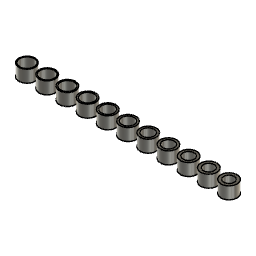
Smartphone inserts generator v4 (Autodesk Fusion 360 design; units mm, degrees)
Autodesk Fusion 360 part; units mm, degrees
sketch "Schizzo1" plane through (0, 0, 0) normal (0, 0, 1) x (1, 0, 0)
  circle A0 centre (0, 0) radius 17.7
  circle A1 centre (0, 0) radius 19.8
  dimension "d2" = 39.6
  dimension "d23" = 35.4
  constraint coincident A0.centre A1.centre
  measures "d2" diameter of A1
  measures "d23" diameter of A0
extrude "Estrusione1" add sketch "Schizzo1" along normal blind 30 makes body 1
pattern_linear "Serie R1" count 11 spacing 50 along (1, 0, 0) of bodies 1 makes body 2 at (69.7016, -1.9714, 20) makes body 3 at (119.7016, -1.9714, 20) makes body 4 at (169.7016, -1.9714, 20) makes body 5 at (219.7016, -1.9714, 20) makes body 6 at (269.7016, -1.9714, 20) makes body 7 at (319.7016, -1.9714, 20) makes body 8 at (369.7016, -1.9714, 20) makes body 9 at (419.7016, -1.9714, 20) makes body 10 at (469.7016, -1.9714, 20) makes body 11 at (510.7424, 16.6325, 20)
move_face "FacceDiOffset2" offset 0.5 1 faces at (67.612, -1.7624, 20) on bodies 2
move_face "FacceDiOffset3" offset 1 1 faces at (117.612, -1.7624, 20) on bodies 3
move_face "FacceDiOffset4" offset 1.5 1 faces at (167.612, -1.7624, 20) on bodies 4
move_face "FacceDiOffset5" offset 2 1 faces at (217.612, -1.7624, 20) on bodies 5
move_face "FacceDiOffset6" offset 2.5 1 faces at (267.612, -1.7624, 20) on bodies 6
move_face "FacceDiOffset7" offset 3 1 faces at (317.612, -1.7624, 20) on bodies 7
move_face "FacceDiOffset8" offset 3.5 1 faces at (367.612, -1.7624, 20) on bodies 8
move_face "FacceDiOffset9" offset 4 1 faces at (417.612, -1.7624, 20) on bodies 9
move_face "FacceDiOffset10" offset 4.5 1 faces at (467.612, -1.7624, 20) on bodies 10
move_face "FacceDiOffset11" offset 5 1 faces at (517.612, -1.7624, 20) on bodies 11
equation "Step = 1 mm"
equation "d13 = Step / 2 * 1"
equation "d14 = Step / 2 * 2"
equation "d15 = Step / 2 * 3"
equation "d16 = Step / 2 * 4"
equation "d17 = Step / 2 * 5"
equation "d18 = Step / 2 * 6"
equation "d19 = Step / 2 * 7"
equation "d20 = Step / 2 * 8"
equation "d21 = Step / 2 * 9"
equation "d22 = Step / 2 * 10"
equation "Start = 35.40 mm"
named bodies: "Insert", "Insert step 1", "Insert step 2", "Insert step 3", "Insert step 4", "Insert step 5", "Insert step 6", "Insert step 7", "Insert step 8", "Insert step 9", "Insert step 10"
